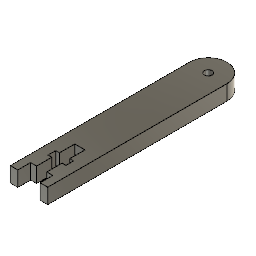
gear_mount v3 (Autodesk Fusion 360 design; units mm, degrees)
Autodesk Fusion 360 part; units mm, degrees
note: some values were not read from the file. Set by a fixed rule: which face or edge a step refers to.
sketch "Sketch1" plane through (0, 0, 0) normal (0, 0, 1) x (1, 0, 0)
  circle A0 centre (0, 0) radius 11
  line L0 (-4.5, 14) -> (4.5, 14)
  line L1 (4.5, 14) -> (4.5, 12)
  line L2 (4.5, 12) -> (-4.5, 12)
  line L3 (-4.5, 12) -> (-4.5, 14)
  line L4 (0, 0) -> (0, 12)
  line L5 (0, 0) -> (11, 0)
  circle A1 centre (0, 0) radius 15.7054
  line L6 (0, 0) -> (-4.5, 14)
  line L7 (-4.5, 14) -> (-4.806, 14.952)
  line L8 (-8.1423, 9.8971) -> (-12.6423, 2.1029)
  line L9 (-14.3744, 3.1029) -> (-9.8744, 10.8971)
  line L10 (-9.8744, 10.8971) -> (-8.1423, 9.8971)
  line L11 (-12.6423, 2.1029) -> (-14.3744, 3.1029)
  line L12 (-12.6423, -2.1029) -> (-8.1423, -9.8971)
  line L13 (-9.8744, -10.8971) -> (-14.3744, -3.1029)
  line L14 (-14.3744, -3.1029) -> (-12.6423, -2.1029)
  line L15 (-8.1423, -9.8971) -> (-9.8744, -10.8971)
  line L16 (-4.5, -12) -> (4.5, -12)
  line L17 (4.5, -14) -> (-4.5, -14)
  line L18 (-4.5, -14) -> (-4.5, -12)
  line L19 (4.5, -12) -> (4.5, -14)
  line L20 (8.1423, -9.8971) -> (12.6423, -2.1029)
  line L21 (14.3744, -3.1029) -> (9.8744, -10.8971)
  line L22 (9.8744, -10.8971) -> (8.1423, -9.8971)
  line L23 (12.6423, -2.1029) -> (14.3744, -3.1029)
  line L24 (12.6423, 2.1029) -> (8.1423, 9.8971)
  line L25 (9.8744, 10.8971) -> (14.3744, 3.1029)
  line L26 (14.3744, 3.1029) -> (12.6423, 2.1029)
  line L27 (8.1423, 9.8971) -> (9.8744, 10.8971)
  circle A2 centre (0, 0) radius 1.25
  line L28 (-4.5, 6.25) -> (4.5, 6.25)
  line L29 (4.5, 6.25) -> (4.5, 2.25)
  line L30 (4.5, 2.25) -> (-4.5, 2.25)
  line L31 (-4.5, 2.25) -> (-4.5, 6.25)
  line L32 (0, 2.25) -> (0, 6.25)
  line L33 (-4.5, 7.25) -> (4.5, 7.25)
  line L34 (5.5, 6.25) -> (5.5, 0)
  line L35 (5.5, 0) -> (-5.5, 0)
  line L36 (-5.5, 0) -> (-5.5, 6.25)
  arc A3 (-4.5, 7.25) -> (-5.5, 6.25) centre (-4.5, 6.25) ccw
  arc A4 (5.5, 6.25) -> (4.5, 7.25) centre (4.5, 6.25) ccw
  line L37 (-5.5, 0) -> (-5.5, -6.25)
  arc A5 (-5.5, -6.25) -> (-4.5, -7.25) centre (-4.5, -6.25) ccw
  line L38 (-4.5, -7.25) -> (4.5, -7.25)
  arc A6 (4.5, -7.25) -> (5.5, -6.25) centre (4.5, -6.25) ccw
  line L39 (5.5, -6.25) -> (5.5, 0)
  line L40 (4.5, -2.25) -> (-4.5, -2.25)
  line L41 (4.5, -6.25) -> (4.5, -2.25)
  line L42 (-4.5, -6.25) -> (4.5, -6.25)
  line L43 (-4.5, -2.25) -> (-4.5, -6.25)
  circle A7 centre (-3.5, 0) radius 1.25
  circle A8 centre (3.5, 0) radius 1.25
  line L44 (-11, 0) -> (-15.7054, 0)
  circle A9 centre (-13.3527, 0) radius 1.25
  circle A10 centre (6.6764, -11.5638) radius 1.25
  circle A11 centre (6.6764, 11.5638) radius 1.25
  point P0 (0, 11)
  point P1 (0, 12)
  point P2 (0, 1.25)
  point P3 (-2.25, 0)
  point P4 (-1.25, 0)
  dimension "d1" = 9
  dimension "d2" = 2
  dimension "d3" = 90
  dimension "d4" = 1
  dimension "d5" = 1
  dimension "d7" = 360
  dimension "d8" = 11
  dimension "d9" = 2.5
  dimension "d10" = 9
  dimension "d11" = 4
  dimension "d12" = 90
  dimension "d13" = 1
  dimension "d14" = 1
  dimension "d15" = 1
  dimension "d16" = 1
  dimension "d17" = 1
  dimension "d18" = 1
  dimension "d19" = 2.5
  dimension "d20" = 1
  dimension "d34" = 2.5
  dimension "d36" = 360
  constraint coincident A0.centre L4.start
  constraint horizontal L0
  constraint vertical L1
  constraint horizontal L2
  constraint vertical L3
  constraint midpoint L2 P1
  constraint coincident A0 L5.end
  constraint parallel L2 L5
  constraint coincident A0 P0
  constraint coincident L4 P0
  constraint coincident P1 L4.end
  constraint concentric A0 A1
  constraint coincident A1 L7.end
  constraint parallel L6 L7
  constraint concentric A1 A2
  constraint horizontal L28
  constraint vertical L29
  constraint horizontal L30
  constraint vertical L31
  constraint midpoint L30 L32.start
  constraint coincident L4 L32.end
  constraint coincident L28 L32.end
  constraint horizontal L33
  constraint vertical L34
  constraint horizontal L35
  constraint vertical L36
  constraint coincident L5 L34.end
  constraint tangent L33 A3
  constraint tangent L36 A3
  constraint tangent L33 A4
  constraint tangent L34 A4
  constraint symmetric L5 L28.start A5.centre
  constraint symmetric L5 L28.end A6.centre
  constraint symmetric L5 L29.end L40.start
  constraint symmetric L5 L30.end L40.end
  constraint symmetric L5 L34.end L35.start
  constraint symmetric L5 L35.end L36.start
  constraint symmetric L5 L33.start A5.end
  constraint symmetric L5 L36.end L37.end
  constraint symmetric L5 A3 A5
  constraint symmetric L5 L33.end L38.end
  constraint symmetric L5 L34.start A6.end
  constraint symmetric L5 A4 A6
  constraint coincident A2 P2
  constraint coincident L4 P2
  constraint coincident L35 A7.centre
  constraint coincident A7 P3
  constraint coincident L35 P3
  constraint coincident A2 P4
  constraint coincident L35 P4
  constraint symmetric L4 A7 A8
  constraint coincident A0 L44.start
  constraint coincident A1 L44.end
  constraint horizontal L44
  constraint midpoint L44 A9.centre
  measures "d1" distance of L0.start L0.end
  measures "d2" distance of L0.start L2.end
  measures "d3" angle of L4 L5
  measures "d4" distance of P0 P1
  measures "d5" distance of L0.start L7.end
  measures "d8" distance of A0.centre L5.end
  measures "d9" diameter of A2
  measures "d10" distance of L28.start L28.end
  measures "d11" distance of L28.start L30.end
  measures "d12" angle of L28 L32
  measures "d13" distance of L31 L36
  measures "d14" distance of L28 L33
  measures "d15" distance of L29 L34
  measures "d16" radius of A3
  measures "d17" radius of A4
  measures "d18" distance of L32.start P2
  measures "d19" diameter of A7
  measures "d20" distance of P3 P4
  measures "d34" diameter of A9
extrude "Extrude1" add sketch "Sketch1" along normal blind 9 contours A0 L2 L3 A1 L6 L7 L44 A9 | A0 L0 L1 L2 L4 A1 L7 L44 A9 | A0 L2 L4 L6 | L5 A2 L35 L37 A5 L38 A6 L39 A7 A8 | L4 L5 A2 L28 L29 L30 L33 L34 L35 A4 A8 | L4 L6 L28 L33 | L6 A2 L28 L30 L31 L33 L35 L36 A3 A7 | L4 L6 A2 L30 makes body 1 at (15.6274, -1.5638, 3) makes body 2 at (5.5, -2.0833, 3)
sketch "Sketch2" plane through (0, 0, 0) normal (0, 0, -1) x (1, 0, 0)
  line L0 (-12.6423, -2.1029) -> (-8.1423, -9.8971)
  line L1 (-8.1423, -9.8971) -> (-9.8744, -10.8971)
  line L2 (-9.8744, -10.8971) -> (-14.3744, -3.1029)
  line L3 (-14.3744, -3.1029) -> (-12.6423, -2.1029)
  line L4 (8.1423, -9.8971) -> (12.6423, -2.1029)
  line L5 (12.6423, -2.1029) -> (14.3744, -3.1029)
  line L6 (14.3744, -3.1029) -> (9.8744, -10.8971)
  line L7 (9.8744, -10.8971) -> (8.1423, -9.8971)
  line L8 (12.6423, 2.1029) -> (8.1423, 9.8971)
  line L9 (8.1423, 9.8971) -> (9.8744, 10.8971)
  line L10 (9.8744, 10.8971) -> (14.3744, 3.1029)
  line L11 (14.3744, 3.1029) -> (12.6423, 2.1029)
  circle A0 centre (0, 0) radius 11
  line L12 (-8.1423, 9.8971) -> (-12.6423, 2.1029)
  line L13 (-12.6423, 2.1029) -> (-14.3744, 3.1029)
  line L14 (-14.3744, 3.1029) -> (-9.8744, 10.8971)
  line L15 (-9.8744, 10.8971) -> (-8.1423, 9.8971)
  line L16 (4.5, 12) -> (-4.5, 12)
  line L17 (-4.5, 12) -> (-4.5, 14)
  line L18 (-4.5, 14) -> (4.5, 14)
  line L19 (4.5, 14) -> (4.5, 12)
  line L20 (-4.5, -12) -> (4.5, -12)
  line L21 (4.5, -12) -> (4.5, -14)
  line L22 (4.5, -14) -> (-4.5, -14)
  line L23 (-4.5, -14) -> (-4.5, -12)
  circle A1 centre (0, 0) radius 15.7054
  circle A2 centre (0, 0) radius 11
  circle A3 centre (0, 0) radius 15.7054
  circle A4 centre (-13.3527, 0) radius 1.25
  circle A5 centre (6.6764, 11.5638) radius 1.25
  circle A6 centre (6.6764, -11.5638) radius 1.25
  constraint concentric A0 A2
  constraint concentric A0 A3
extrude "Extrude2" add sketch "Sketch2" along normal blind 1 contours L0 L1 L2 L3 | L4 L5 L6 L7 | L8 L9 L10 L11 | L12 L13 L14 L15 | L16 L17 L18 L19 | L20 L21 L22 L23 | A1 A3 | A4 | A5 | A6 bodies 1
sketch "Sketch3" plane through (0, 0, 0) normal (0, 0, -1) x (1, 0, 0)
  line L0 (-4.5, 2.25) -> (-4.5, 6.25)
  line L1 (-4.5, 6.25) -> (4.5, 6.25)
  line L2 (4.5, 6.25) -> (4.5, 2.25)
  line L3 (4.5, 2.25) -> (-4.5, 2.25)
  circle A0 centre (3.5, 0) radius 1.25
  circle A1 centre (-3.5, 0) radius 1.25
  line L4 (-4.5, -2.25) -> (4.5, -2.25)
  line L5 (4.5, -2.25) -> (4.5, -6.25)
  line L6 (4.5, -6.25) -> (-4.5, -6.25)
  line L7 (-4.5, -6.25) -> (-4.5, -2.25)
  circle A2 centre (0, 0) radius 1.25
  line L8 (-5.5, 6.25) -> (-5.5, -6.25)
  arc A3 (-5.5, -6.25) -> (-4.5, -7.25) centre (-4.5, -6.25) ccw
  line L9 (-4.5, -7.25) -> (4.5, -7.25)
  arc A4 (4.5, -7.25) -> (5.5, -6.25) centre (4.5, -6.25) ccw
  line L10 (5.5, -6.25) -> (5.5, 6.25)
  arc A5 (5.5, 6.25) -> (4.5, 7.25) centre (4.5, 6.25) ccw
  line L11 (4.5, 7.25) -> (-4.5, 7.25)
  arc A6 (-4.5, 7.25) -> (-5.5, 6.25) centre (-4.5, 6.25) ccw
  line L12 (-6, 8) -> (6, 8)
  line L13 (6, 8) -> (6, -8)
  line L14 (6, -8) -> (-6, -8)
  line L15 (-6, -8) -> (-6, 8)
  constraint horizontal L12
  constraint vertical L13
  constraint horizontal L14
  constraint vertical L15
extrude "Extrude3" add sketch "Sketch3" along normal blind 1 contours L0 L1 L2 L3 | L4 L5 L6 L7 | L8 A3 L9 A4 L10 A5 L11 A6 bodies 2
sketch "Sketch4" plane through (0, 0, -1) normal (0, 0, -1) x (1, 0, 0)
  circle A0 centre (0, 0) radius 11
  circle A1 centre (0, 0) radius 15.7054
  line L0 (0, 0) -> (12.1661, 12.1661)
  circle A2 centre (12.1661, 12.1661) radius 1.5
  line L1 (0, 0) -> (11, 0)
  circle A3 centre (12.1661, 12.1661) radius 2.5
  line L2 (5.6184, 14.6661) -> (14.047, 14.6661)
  line L3 (14.6661, 5.6184) -> (14.6661, 14.047)
  line L4 (-14.6661, 5.6184) -> (-14.6661, 14.047)
  circle A4 centre (-12.1661, 12.1661) radius 2.5
  line L5 (-5.6184, 14.6661) -> (-14.047, 14.6661)
  circle A5 centre (-12.1661, 12.1661) radius 1.5
  line L6 (-5.6184, -14.6661) -> (-14.047, -14.6661)
  circle A6 centre (-12.1661, -12.1661) radius 2.5
  line L7 (-14.6661, -5.6184) -> (-14.6661, -14.047)
  circle A7 centre (-12.1661, -12.1661) radius 1.5
  line L8 (14.6661, -5.6184) -> (14.6661, -14.047)
  circle A8 centre (12.1661, -12.1661) radius 2.5
  line L9 (5.6184, -14.6661) -> (14.047, -14.6661)
  circle A9 centre (12.1661, -12.1661) radius 1.5
  dimension "d27" = 3
  dimension "d28" = 45
  dimension "d29" = 1
  dimension "d31" = 360
  constraint coincident A0.centre A1.centre
  constraint coincident L0.end A2.centre
  constraint tangent A1 A2
  constraint coincident A0 L1.end
  constraint horizontal L1
  constraint coincident A1 L2.start
  constraint tangent A3 L2
  constraint horizontal L2
  constraint symmetric L0 L2.start L3.start
  constraint symmetric L0 L2.end L3.end
  measures "d27" diameter of A2
  measures "d28" angle of L0 L1
extrude "Extrude4" add sketch "Sketch4" against normal blind 2 contours A1 A3 L3 | A1 L8 A8 | A1 A3 | A1 A8 | A1 A3 L2 | A1 A8 L9 | A1 A4 L5 | A1 L6 A6 | A1 A4 | A1 A6 | A1 L4 A4 | A1 A6 L7 picked at (10.2026, -12.4068) picked at (-10.1946, 12.3655) picked at (-10.1946, -12.3655) bodies 1
extrude "Extrude5" cut 3 faces at (-12.9857, 0.2927, 0) (7.0003, -11.97, 0) (7.0345, 11.8592, 0) along direction (0, 0, -1) blind 3 on bodies 1 bodies 1
sketch "Sketch5" plane through (14.6661, 0, 0) normal (1, 0, 0) x (0, 1, 0)
  line L0 (-12.1661, -1) -> (-5.6184, -1)
  line L1 (-5.6184, -1) -> (-5.6184, 1)
  line L2 (-5.6184, 1) -> (-12.1661, 1)
  line L3 (-12.1661, 1) -> (-12.1661, -1)
  line L4 (-18.8545, 1) -> (17, 1)
  line L5 (17, 1) -> (17, 12)
  line L6 (17, 12) -> (-18.8545, 12)
  line L7 (-18.8545, 12) -> (-18.8545, 1)
  constraint horizontal L4
  constraint vertical L5
  constraint horizontal L6
  constraint vertical L7
extrude "Extrude6" cut sketch "Sketch5" against normal blind 100 from surface at 10 contours L2 L4 L5 L6 L7 bodies 2 1
extrude "Extrude7" cut 1 faces at (0.0311, 5.2488, -1) along direction (0, 0, 1) blind 10 on bodies 2 bodies 2
sketch "Sketch6" plane through (0, 0, -1) normal (0, 0, -1) x (1, 0, 0)
  circle A0 centre (6.6764, 11.5638) radius 1.25
  circle A1 centre (-13.3527, 0) radius 1.25
  circle A2 centre (6.6764, -11.5638) radius 1.25
  circle A3 centre (12.1661, 12.1661) radius 1.5
  circle A4 centre (-12.1661, 12.1661) radius 1.5
  circle A5 centre (12.1661, -12.1661) radius 1.5
  circle A6 centre (-12.1661, -12.1661) radius 1.5
  circle A7 centre (0, 0) radius 11
  line L0 (14.6661, 5.6184) -> (14.6661, 12.1661)
  arc A8 (14.6661, 12.1661) -> (12.1661, 14.6661) centre (12.1661, 12.1661) ccw
  line L1 (12.1661, 14.6661) -> (5.6184, 14.6661)
  arc A9 (5.6184, 14.6661) -> (-5.6184, 14.6661) centre (0, 0) ccw
  line L2 (-5.6184, 14.6661) -> (-12.1661, 14.6661)
  arc A10 (-12.1661, 14.6661) -> (-14.6661, 12.1661) centre (-12.1661, 12.1661) ccw
  line L3 (-14.6661, 12.1661) -> (-14.6661, 5.6184)
  arc A11 (-14.6661, 5.6184) -> (-14.6661, -5.6184) centre (0, 0) ccw
  line L4 (-14.6661, -5.6184) -> (-14.6661, -12.1661)
  arc A12 (-14.6661, -12.1661) -> (-12.1661, -14.6661) centre (-12.1661, -12.1661) ccw
  line L5 (-12.1661, -14.6661) -> (-5.6184, -14.6661)
  arc A13 (-5.6184, -14.6661) -> (5.6184, -14.6661) centre (0, 0) ccw
  line L6 (5.6184, -14.6661) -> (12.1661, -14.6661)
  arc A14 (12.1661, -14.6661) -> (14.6661, -12.1661) centre (12.1661, -12.1661) ccw
  line L7 (14.6661, -12.1661) -> (14.6661, -5.6184)
  arc A15 (14.6661, -5.6184) -> (14.6661, 5.6184) centre (0, 0) ccw
  circle A16 centre (0, 0) radius 10.35
  line L8 (-7.0258, 7.6) -> (7.0258, 7.6)
  line L9 (0, 0) -> (10.35, 0)
  line L10 (-7.0258, -7.6) -> (7.0258, -7.6)
  circle A17 centre (0, 0) radius 12.1027
  line L11 (-7.3699, 9.6) -> (7.3699, 9.6)
  line L12 (-7.3699, -9.6) -> (7.3699, -9.6)
  dimension "d44" = 20.7
  dimension "d47" = 2
  dimension "d56" = 7.6
  constraint coincident A7.centre A9.centre
  constraint coincident A16 L8.start
  constraint coincident A16 L8.end
  constraint horizontal L8
  constraint coincident A16 L9.end
  constraint horizontal L9
  constraint symmetric L8.start L9 L10.start
  constraint symmetric L8.end L9 L10.end
  constraint concentric A16 A17
  constraint coincident A17 L11.start
  constraint coincident A17 L11.end
  constraint horizontal L11
  constraint symmetric L9 L11.start L12.start
  constraint symmetric L9 L11.end L12.end
  constraint tangent A1 A17
  measures "d44" diameter of A16
  measures "d47" distance of L8 L11
  measures "d56" distance of L8 A7.centre
extrude "Extrude8" add sketch "Sketch6" along normal blind 10 from surface at -2 contours A7 A17 L11 L12 | A7 A17 L11 L12 | A7 A16 L11 L12 | A7 A16 L11 L12 | A16 L8 L11 | A16 L10 L12 bodies 1 2
extrude "Extrude9" add sketch "Sketch6" along normal up to surface (2 mm away) from surface at -2 contours A7 A16 L11 | A16 L11 | A7 A16 L12 | A16 L12 bodies 1
extrude "Extrude10" add 6 faces at (11.4857, -6.8337, 0) (11.661, 6.5301, 0) (-1.5, 12.6667, 0) (-11.4857, 6.8337, 0) (-11.661, -6.5301, 0) (1.5, -12.6667, 0) along direction (0, 0, 1) up to surface end surface through (24.6661, -5.6184, 1) normal (0, 0, 1) offset 0 on bodies 1 bodies 1
extrude "Extrude11" add 5 faces at (6.0368, -9.6, -3.6667) (-6.0368, -9.6, -6.3333) (4.8696, -9.6, -6.3333) (-1.2894, -9.6, -3.6667) (-4.8696, -9.6, -3.6667) along direction (0, -1, 0) blind 20 start surface through (-5.6184, -14.6661, -1) normal (0, -1, 0) on bodies 1 bodies 1
extrude "Extrude12" add 1 faces at (1.8728, -14.6661, -6.3333) along direction (0, 1, 0) up to surface (5.0661 mm away) on bodies 1 bodies 1
extrude "Extrude13" add 1 faces at (0.3827, -28.3319, -1) along direction (0, 0, 1) up to surface (2 mm away) on bodies 1 bodies 1
sketch "Sketch7" plane through (0, 0, 1) normal (0, 0, 1) x (-1, 0, 0)
  arc A0 (7.0258, -7.6) -> (7.0258, 7.6) centre (0, 0) ccw
  line L0 (7.0258, -7.6) -> (-7.0258, -7.6)
  arc A1 (-7.0258, 7.6) -> (-7.0258, -7.6) centre (0, 0) ccw
  line L1 (-7.0258, 7.6) -> (7.0258, 7.6)
  circle A2 centre (13.3527, 0) radius 1.25
  arc A3 (-14.6661, 5.6184) -> (-14.6661, -5.6184) centre (0, 0) ccw
  line L2 (-14.6661, -5.6184) -> (-14.6661, -12.1661)
  arc A4 (-14.6661, -12.1661) -> (-12.1661, -14.6661) centre (-12.1661, -12.1661) ccw
  line L3 (-12.1661, -14.6661) -> (-5.6184, -14.6661)
  arc A5 (-5.6184, -14.6661) -> (5.6184, -14.6661) centre (0, 0) ccw
  line L4 (5.6184, -14.6661) -> (12.1661, -14.6661)
  arc A6 (12.1661, -14.6661) -> (14.6661, -12.1661) centre (12.1661, -12.1661) ccw
  line L5 (14.6661, -12.1661) -> (14.6661, -5.6184)
  arc A7 (14.6661, -5.6184) -> (14.6661, 5.6184) centre (0, 0) ccw
  line L6 (14.6661, 5.6184) -> (14.6661, 12.1661)
  arc A8 (14.6661, 12.1661) -> (12.1661, 14.6661) centre (12.1661, 12.1661) ccw
  line L7 (12.1661, 14.6661) -> (7.3699, 14.6661)
  line L8 (7.3699, 14.6661) -> (7.3699, 34.6661)
  line L9 (7.3699, 34.6661) -> (-7.3699, 34.6661)
  line L10 (-7.3699, 34.6661) -> (-7.3699, 14.6661)
  line L11 (-7.3699, 14.6661) -> (-12.1661, 14.6661)
  arc A9 (-12.1661, 14.6661) -> (-14.6661, 12.1661) centre (-12.1661, 12.1661) ccw
  line L12 (-14.6661, 12.1661) -> (-14.6661, 5.6184)
  circle A10 centre (12.1661, 12.1661) radius 1.5
  circle A11 centre (12.1661, -12.1661) radius 1.5
  circle A12 centre (-6.6764, 11.5638) radius 1.25
  circle A13 centre (-6.6764, -11.5638) radius 1.25
  circle A14 centre (-12.1661, -12.1661) radius 1.5
  circle A15 centre (-12.1661, 12.1661) radius 1.5
  circle A16 centre (-6.6764, 11.5638) radius 1.25
  constraint concentric A12 A16
extrude "Extrude14" add sketch "Sketch7" against normal blind 2 contours A12 A16 bodies 1
sketch "Sketch8" plane through (0, 0, 1) normal (0, 0, 1) x (-1, 0, 0)
  arc A0 (7.0258, -7.6) -> (7.0258, 7.6) centre (0, 0) ccw
  line L0 (7.0258, -7.6) -> (-7.0258, -7.6)
  arc A1 (-7.0258, 7.6) -> (-7.0258, -7.6) centre (0, 0) ccw
  line L1 (-7.0258, 7.6) -> (7.0258, 7.6)
  circle A2 centre (13.3527, 0) radius 1.25
  arc A3 (-14.6661, 5.6184) -> (-14.6661, -5.6184) centre (0, 0) ccw
  line L2 (-14.6661, -5.6184) -> (-14.6661, -12.1661)
  arc A4 (-14.6661, -12.1661) -> (-12.1661, -14.6661) centre (-12.1661, -12.1661) ccw
  line L3 (-12.1661, -14.6661) -> (-5.6184, -14.6661)
  arc A5 (-5.6184, -14.6661) -> (5.6184, -14.6661) centre (0, 0) ccw
  line L4 (5.6184, -14.6661) -> (12.1661, -14.6661)
  arc A6 (12.1661, -14.6661) -> (14.6661, -12.1661) centre (12.1661, -12.1661) ccw
  line L5 (14.6661, -12.1661) -> (14.6661, -5.6184)
  arc A7 (14.6661, -5.6184) -> (14.6661, 5.6184) centre (0, 0) ccw
  line L6 (14.6661, 5.6184) -> (14.6661, 12.1661)
  arc A8 (14.6661, 12.1661) -> (12.1661, 14.6661) centre (12.1661, 12.1661) ccw
  line L7 (12.1661, 14.6661) -> (7.3699, 14.6661)
  line L8 (7.3699, 14.6661) -> (7.3699, 34.6661)
  line L9 (7.3699, 34.6661) -> (-7.3699, 34.6661)
  line L10 (-7.3699, 34.6661) -> (-7.3699, 14.6661)
  line L11 (-7.3699, 14.6661) -> (-12.1661, 14.6661)
  arc A9 (-12.1661, 14.6661) -> (-14.6661, 12.1661) centre (-12.1661, 12.1661) ccw
  line L12 (-14.6661, 12.1661) -> (-14.6661, 5.6184)
  circle A10 centre (12.1661, 12.1661) radius 1.5
  circle A11 centre (12.1661, -12.1661) radius 1.5
  circle A12 centre (-6.6764, -11.5638) radius 1.25
  circle A13 centre (-12.1661, -12.1661) radius 1.5
  circle A14 centre (-12.1661, 12.1661) radius 1.5
  line L13 (2, 34.6661) -> (-2, 34.6661)
  line L14 (-2, 34.6661) -> (-2, 19.6661)
  line L15 (-2, 19.6661) -> (2, 19.6661)
  line L16 (2, 19.6661) -> (2, 34.6661)
  line L17 (0, 19.6661) -> (0, 34.6661)
  line L18 (3.5, 25.6661) -> (-3.5, 25.6661)
  line L19 (-3.5, 25.6661) -> (-3.5, 28.6661)
  line L20 (-3.5, 28.6661) -> (3.5, 28.6661)
  line L21 (3.5, 28.6661) -> (3.5, 25.6661)
  line L22 (0, 34.6661) -> (0, 28.6661)
  line L23 (3.5, 27.1661) -> (0, 27.1661)
  dimension "d66" = 4
  dimension "d68" = 90
  dimension "d69" = 15
  dimension "d70" = 7
  dimension "d71" = 3
  dimension "d72" = 90
  dimension "d73" = 90
  constraint horizontal L13
  constraint vertical L14
  constraint horizontal L15
  constraint vertical L16
  constraint coincident L9 L13.start
  constraint midpoint L15 L17.start
  constraint midpoint L9 L17.end
  constraint horizontal L18
  constraint vertical L19
  constraint horizontal L20
  constraint vertical L21
  constraint midpoint L20 L22.end
  constraint midpoint L21 L23.start
  constraint midpoint L17 L23.end
  measures "d66" distance of L14.end L15.end
  measures "d68" angle of L9 L17
  measures "d69" distance of L13.end L14.end
  measures "d70" distance of L19.end L20.end
  measures "d71" distance of L18.end L19.end
  measures "d72" angle of L20 L22
  measures "d73" angle of L17 L23
extrude "Extrude15" cut sketch "Sketch8" against normal blind 100 contours L9 L13 L14 L17 L20 L22 | L9 L13 L16 L17 L20 L22 | L14 L17 L18 L20 | L14 L18 L19 L20 | L16 L17 L20 L23 | L14 L15 L17 L18 | L16 L20 L21 L23 | L16 L17 L18 L23 | L15 L16 L17 L18 | L16 L18 L21 L23 bodies 1
sketch "Sketch9" plane through (0, -34.6661, 0) normal (0, -1, 0) x (1, 0, 0)
  line L0 (-2, -9) -> (-2, 1)
  line L1 (-2, 1) -> (-7.3699, 1)
  line L2 (-7.3699, 1) -> (-7.3699, -9)
  line L3 (-7.3699, -9) -> (-2, -9)
  line L4 (-7.3699, 1) -> (-4.3699, 1)
  line L5 (-4.3699, 1) -> (-4.3699, -9)
  line L6 (-4.3699, -9) -> (-7.3699, -9)
  line L7 (-7.3699, -9) -> (-7.3699, 1)
  dimension "d76" = 3
  constraint horizontal L4
  constraint vertical L5
  constraint horizontal L6
  constraint vertical L7
  constraint coincident L3 L5.end
  constraint coincident L1.end L2.start
  measures "d76" distance of L1.end L4.end
extrude "Extrude16" add sketch "Sketch9" along normal blind 5 contours L1 L2 L3 L4 L5 L6 L7 bodies 1
sketch "Sketch10" plane through (0, -34.6661, 0) normal (0, -1, 0) x (1, 0, 0)
  line L0 (2, 1) -> (2, -9)
  line L1 (2, -9) -> (7.3699, -9)
  line L2 (7.3699, -9) -> (7.3699, 1)
  line L3 (7.3699, 1) -> (2, 1)
  line L4 (7.3699, 1) -> (4.3699, 1)
  line L5 (4.3699, 1) -> (4.3699, -9)
  line L6 (4.3699, -9) -> (7.3699, -9)
  line L7 (7.3699, -9) -> (7.3699, 1)
  dimension "d79" = 3
  constraint horizontal L4
  constraint vertical L5
  constraint horizontal L6
  constraint vertical L7
  constraint coincident L1 L5.end
  constraint coincident L2.end L3.start
  measures "d79" distance of L2.end L4.end
extrude "Extrude17" add sketch "Sketch10" along normal blind 5 contours L1 L2 L3 L4 L5 L6 L7 bodies 1
extrude "Extrude18" cut 1 faces at (2.3419, -12.3107, 1) along direction (0, 0, -1) blind 4 on bodies 1 bodies 1
sketch "Sketch11" plane through (0, 0, -3) normal (0, 0, 1) x (-1, 0, 0)
  line L0 (-7.3699, 39.6661) -> (-7.3699, 9.6)
  arc A0 (-7.3699, 9.6) -> (-7.3699, -9.6) centre (0, 0) ccw
  line L1 (-7.3699, -9.6) -> (7.3699, -9.6)
  arc A1 (7.3699, -9.6) -> (7.3699, 9.6) centre (0, 0) ccw
  line L2 (7.3699, 9.6) -> (7.3699, 39.6661)
  line L3 (7.3699, 39.6661) -> (4.3699, 39.6661)
  line L4 (4.3699, 39.6661) -> (4.3699, 34.6661)
  line L5 (4.3699, 34.6661) -> (2, 34.6661)
  line L6 (2, 34.6661) -> (2, 28.6661)
  line L7 (2, 28.6661) -> (3.5, 28.6661)
  line L8 (3.5, 28.6661) -> (3.5, 25.6661)
  line L9 (3.5, 25.6661) -> (2, 25.6661)
  line L10 (2, 25.6661) -> (2, 19.6661)
  line L11 (2, 19.6661) -> (-2, 19.6661)
  line L12 (-2, 19.6661) -> (-2, 25.6661)
  line L13 (-2, 25.6661) -> (-3.5, 25.6661)
  line L14 (-3.5, 25.6661) -> (-3.5, 28.6661)
  line L15 (-3.5, 28.6661) -> (-2, 28.6661)
  line L16 (-2, 28.6661) -> (-2, 34.6661)
  line L17 (-2, 34.6661) -> (-4.3699, 34.6661)
  line L18 (-4.3699, 34.6661) -> (-4.3699, 39.6661)
  line L19 (-4.3699, 39.6661) -> (-7.3699, 39.6661)
  arc A2 (7.0258, -7.6) -> (7.0258, 7.6) centre (0, 0) ccw
  line L20 (7.0258, -7.6) -> (-7.0258, -7.6)
  arc A3 (-7.0258, 7.6) -> (-7.0258, -7.6) centre (0, 0) ccw
  line L21 (-7.0258, 7.6) -> (7.0258, 7.6)
  line L22 (25, 14.6661) -> (-22, 14.6661)
  line L23 (-22, 14.6661) -> (-22, -14.9245)
  line L24 (-22, -14.9245) -> (25, -14.9245)
  line L25 (25, -14.9245) -> (25, 14.6661)
  dimension "d84" = 25
  constraint horizontal L22
  constraint vertical L23
  constraint horizontal L24
  constraint vertical L25
  measures "d84" distance of L2.end L22
extrude "Extrude19" cut sketch "Sketch11" against normal blind 100 contours L0 A0 L1 A1 L2 L22 bodies 1
sketch "Sketch12" plane through (0, 0, -3) normal (0, 0, 1) x (-1, 0, 0)
  line L0 (-7.3699, 14.6661) -> (7.3699, 14.6661)
  line L1 (7.3699, 14.6661) -> (7.3699, 39.6661)
  line L2 (7.3699, 39.6661) -> (4.3699, 39.6661)
  line L3 (4.3699, 39.6661) -> (4.3699, 34.6661)
  line L4 (4.3699, 34.6661) -> (2, 34.6661)
  line L5 (2, 34.6661) -> (2, 28.6661)
  line L6 (2, 28.6661) -> (3.5, 28.6661)
  line L7 (3.5, 28.6661) -> (3.5, 25.6661)
  line L8 (3.5, 25.6661) -> (2, 25.6661)
  line L9 (2, 25.6661) -> (2, 19.6661)
  line L10 (2, 19.6661) -> (-2, 19.6661)
  line L11 (-2, 19.6661) -> (-2, 25.6661)
  line L12 (-2, 25.6661) -> (-3.5, 25.6661)
  line L13 (-3.5, 25.6661) -> (-3.5, 28.6661)
  line L14 (-3.5, 28.6661) -> (-2, 28.6661)
  line L15 (-2, 28.6661) -> (-2, 34.6661)
  line L16 (-2, 34.6661) -> (-4.3699, 34.6661)
  line L17 (-4.3699, 34.6661) -> (-4.3699, 39.6661)
  line L18 (-4.3699, 39.6661) -> (-7.3699, 39.6661)
  line L19 (-7.3699, 39.6661) -> (-7.3699, 14.6661)
  line L20 (7.3699, 14.6661) -> (-7.3699, 14.6661)
  line L21 (-7.3699, 14.6661) -> (-7.3699, -30.7239)
  line L22 (-7.3699, -30.7239) -> (7.3699, -30.7239)
  line L23 (7.3699, -30.7239) -> (7.3699, 14.6661)
  line L24 (7.3699, -30.7239) -> (-7.3699, -30.7239)
  line L25 (-7.3699, -30.7239) -> (-7.3699, -46.856)
  line L26 (-7.3699, -46.856) -> (7.3699, -46.856)
  line L27 (7.3699, -46.856) -> (7.3699, -30.7239)
  line L28 (0, -30.7239) -> (0, -46.856)
  circle A0 centre (0, -30.7239) radius 1.5
  circle A1 centre (0, -30.7239) radius 7.3699
  dimension "d87" = 65.39
  dimension "d88" = 3
  constraint horizontal L20
  constraint vertical L21
  constraint horizontal L22
  constraint vertical L23
  constraint coincident L0.end L1.start
  constraint horizontal L24
  constraint vertical L25
  constraint horizontal L26
  constraint vertical L27
  constraint midpoint L22 L28.start
  constraint midpoint L26 L28.end
  constraint perpendicular L26 L28
  constraint coincident L28.start A0.centre
  constraint concentric A0 A1
  constraint coincident L22.end A1
  measures "d87" distance of L16 L22
  measures "d88" diameter of A0
extrude "Extrude20" add sketch "Sketch12" against normal up to surface (6 mm away) contours L0 L20 L21 L23 A1 | L22 L24 A0 A1 | L22 L24 L28 A0 A1 | L22 L24 L28 A0 A1 bodies 1
